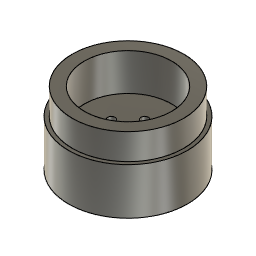
Felge_2.0 v2 (Autodesk Fusion 360 design; units mm, degrees)
Autodesk Fusion 360 part; units mm, degrees
sketch "Skizze2" plane through (0, 0, 0) normal (0, 0, 1) x (1, 0, 0)
  circle A0 centre (0, 0) radius 16
  dimension "d2" = 32
  constraint coincident A0.centre origin
  measures "d2" diameter of A0
extrude "Extrusion1" add sketch "Skizze2" along normal blind 12.5
sketch "Skizze3" plane through (0, 0, 12.5) normal (0, 0, 1) x (-1, 0, 0)
  circle A0 centre (0, 0) radius 16
  circle A1 centre (0, 0) radius 15
  dimension "d5" = 30
  constraint coincident A0.centre A1.centre
  measures "d5" diameter of A1
extrude "Extrusion2" add sketch "Skizze3" along normal blind 7 contours A1
sketch "Skizze4" plane through (0, 0, 19.5) normal (0, 0, 1) x (-1, 0, 0)
  circle A0 centre (0, 0) radius 15
  circle A1 centre (0, 0) radius 11.75
  dimension "d8" = 23.5
  constraint coincident A0.centre A1.centre
  measures "d8" diameter of A1
extrude "Extrusion3" cut sketch "Skizze4" against normal blind 10 contours A1
sketch "Skizze5" plane through (0, 0, 9.5) normal (0, 0, 1) x (-1, 0, 0)
  circle A0 centre (0, 0) radius 11.75
  circle A1 centre (0, 0) radius 1.15
  dimension "d11" = 2.3
  constraint coincident A0.centre A1.centre
  measures "d11" diameter of A1
extrude "Extrusion4" cut sketch "Skizze5" against normal blind 300 contours A1
sketch "Skizze6" plane through (0, 0, 0) normal (0, 0, -1) x (1, 0, 0)
  circle A0 centre (0, 0) radius 1.15
  circle A1 centre (0, 0) radius 16
  circle A2 centre (0, 0) radius 12.5
  dimension "d14" = 25
  constraint coincident A0.centre A1.centre
  measures "d14" diameter of A2
extrude "Extrusion5" cut sketch "Skizze6" against normal blind 5 contours A2
sketch "Skizze7" plane through (0, 0, 5) normal (0, 0, -1) x (1, 0, 0)
  circle A0 centre (0, 0) radius 1.15
  circle A1 centre (0, 0) radius 12.5
  circle A2 centre (0, -4.5) radius 1
  dimension "d17" = 2
  measures "d17" diameter of A2
extrude "Extrusion6" cut sketch "Skizze7" against normal blind 300 contours A2
sketch "Skizze8" plane through (0, 0, 5) normal (0, 0, -1) x (1, 0, 0)
  circle A0 centre (0, -4.5) radius 1
  circle A1 centre (0, 0) radius 1.15
  circle A2 centre (0, 0) radius 12.5
  circle A3 centre (4.5, 0) radius 1
  dimension "d20" = 2
  measures "d20" diameter of A3
extrude "Extrusion7" cut sketch "Skizze8" against normal blind 300 contours A3
sketch "Skizze9" plane through (0, 0, 5) normal (0, 0, -1) x (1, 0, 0)
  circle A0 centre (4.5, 0) radius 1
  circle A1 centre (0, -4.5) radius 1
  circle A2 centre (0, 0) radius 1.15
  circle A3 centre (0, 0) radius 12.5
  circle A4 centre (0, 4.5) radius 1
  dimension "d23" = 2
  measures "d23" diameter of A4
extrude "Extrusion8" cut sketch "Skizze9" against normal blind 300 contours A4
sketch "Skizze10" plane through (0, 0, 5) normal (0, 0, -1) x (1, 0, 0)
  circle A0 centre (0, 4.5) radius 1
  circle A1 centre (4.5, 0) radius 1
  circle A2 centre (0, -4.5) radius 1
  circle A3 centre (0, 0) radius 1.15
  circle A4 centre (0, 0) radius 12.5
  circle A5 centre (-4.5, 0) radius 1
  dimension "d26" = 2
  measures "d26" diameter of A5
extrude "Extrusion9" cut sketch "Skizze10" against normal blind 300 contours A5
